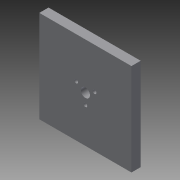
# Autodesk Inventor part: 5_16_18_tee_nut
Saved by Autodesk Inventor 2014 (Build 180170000, 170)
## iProperties
Created: 2015-03-09
Part Number: 5_16_18_tee_nut
Material: Generic
Document SubType Name: Modeling
Designer: cruiser
Density: 1 g/cm^3
Appearance: Default
Author: cruiser
Autodesk Inventor part; units mm, degrees
ref_plane "YZ Plane" through (0, 0, 0) normal (1, 0, 0) x (0, 1, 0)
ref_plane "XZ Plane" through (0, 0, 0) normal (0, 1, 0) x (-1, 0, 0)
ref_plane "XY Plane" through (0, 0, 0) normal (0, 0, 1) x (1, 0, 0)
sketch "Sketch1" plane through (0, 0, 0) normal (0, 1, 0) x (-1, 0, 0)
  line L0 (50, -50) -> (-50, -50)
  line L1 (-50, -50) -> (-50, 50)
  line L2 (-50, 50) -> (50, 50)
  line L3 (50, 50) -> (50, -50)
  line L4 (50, -50) -> (-50, 50) construction
  line L5 (-50, -50) -> (50, 50) construction
  point P0 (0, 0)
  dimension "d0" = 100
  dimension "d1" = 100
  constraints: 12 end point, 2 midpoint, 2 parallel, 1 horizontal, 1 perpendicular
  measures "d0" distance of L1.end L2.end
  measures "d1" distance of L0.end L1.end
extrude "Extrusion1" add sketch "Sketch1" along normal blind 10
sketch "Sketch2" plane through (0, 10, 0) normal (0, 1, 0) x (1, 0, 0)
  circle A0 centre (0, 0) radius 5
  line L0 (0, 0) -> (0, 11.5062)
  circle A1 centre (0, 11.5062) radius 2
  circle A2 centre (-9.9647, -5.7531) radius 2
  circle A3 centre (9.9647, -5.7531) radius 2
  line L1 (0, 0) -> (0, 14.6522)
  dimension "center_hole" = 10
  dimension "d5" = 11.5062
  dimension "hole" = 4
  dimension "d9" = 360
  dimension "d13" = 0
  constraints: 4 centre point, 4 end point, 2 coincident, 1 vertical, 7 other
  measures "center_hole" diameter of A0
  measures "d5" distance of L0.start L0.end
  measures "hole" diameter of A1
  measures "d13" distance between parallel lines of L0 L1
extrude "Extrusion2" cut sketch "Sketch2" against normal up to next
body "Solid1"
